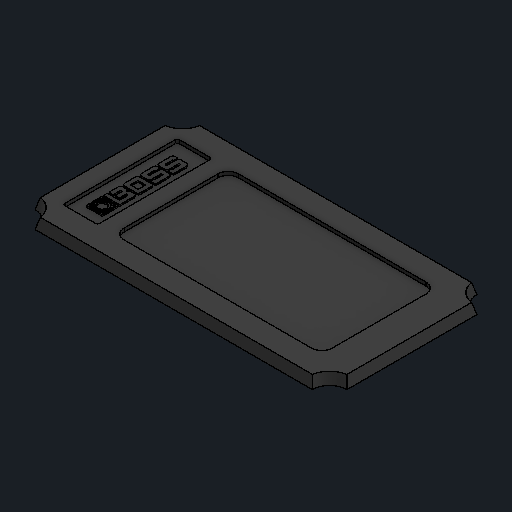
# Autodesk Inventor part: Bottom
Saved by Autodesk Inventor 2026.2 (Build 302298000, 298)
## iProperties
Created: 2015-05-06
Part Number: Bottom
Material: Rubber
Document SubType Name: Modeling
Designer: Philip
Density: 0.93 g/cm^3
Appearance: Rubber - Black
Author: Philip
Autodesk Inventor part; units mm, degrees
(part 1 of 2)
ref_plane "YZ Plane" through (0, 0, 0) normal (1, 0, 0) x (0, 1, 0)
ref_plane "XZ Plane" through (0, 0, 0) normal (0, 1, 0) x (-1, 0, 0)
ref_plane "XY Plane" through (0, 0, 0) normal (0, 0, 1) x (1, 0, 0)
sketch "Sketch1" plane through (0, 0, 0) normal (0, 1, 0) x (-1, 0, 0)
  line L0 (-50.8, 30.1625) -> (50.8, 30.1625)
  line L1 (57.15, 23.8125) -> (57.15, -23.8125)
  line L2 (50.8, -30.1625) -> (-50.8, -30.1625)
  line L3 (-57.15, -23.8125) -> (-57.15, 23.8125)
  arc A0 (57.15, -23.8125) -> (50.8, -30.1625) centre (57.15, -30.1625) ccw
  arc A1 (50.8, 30.1625) -> (57.15, 23.8125) centre (57.15, 30.1625) ccw
  arc A2 (-57.15, 23.8125) -> (-50.8, 30.1625) centre (-57.15, 30.1625) ccw
  arc A3 (-50.8, -30.1625) -> (-57.15, -23.8125) centre (-57.15, -30.1625) ccw
  point P0 (0, 0)
  dimension "d2" = 30.1625
  dimension "d3" = 57.15
  dimension "d4" = 12.7
  dimension "d5" = 12.7
  dimension "d6" = 12.7
  dimension "d7" = 12.7
  dimension "d8" = 60.325
  dimension "d9" = 114.3
  constraints: 8 end point, 8 point on circle, 8 point on line, 4 centre point, 2 parallel, 1 horizontal, 1 perpendicular
  measures "d2" distance from line of L2 point (0, 0)
  measures "d3" distance from line of L3 point (0, 0)
  measures "d4" diameter of A1
  measures "d5" diameter of A0
  measures "d6" diameter of A3
  measures "d7" diameter of A2
  measures "d8" distance between parallel lines of L0 L2
  measures "d9" distance between parallel lines of L3 L1
extrude "Extrusion1" add sketch "Sketch1" along normal blind 3.81 draft -15
sketch "Sketch2" plane through (0, 3.81, 0) normal (0, 1, 0) x (1, 0, 0)
  line L0 (41.275, -20.955) -> (-27.305, -20.955)
  line L1 (-31.115, -17.145) -> (-31.115, 17.145)
  line L2 (-27.305, 20.955) -> (41.275, 20.955)
  line L3 (45.085, 17.145) -> (45.085, -17.145)
  line L4 (57.15, -23.8125) -> (57.15, 23.8125) projected
  arc A0 (-31.115, -17.145) -> (-27.305, -20.955) centre (-27.305, -17.145) ccw
  arc A1 (-27.305, 20.955) -> (-31.115, 17.145) centre (-27.305, 17.145) ccw
  arc A2 (45.085, 17.145) -> (41.275, 20.955) centre (41.275, 17.145) ccw
  arc A3 (41.275, -20.955) -> (45.085, -17.145) centre (41.275, -17.145) ccw
  point P0 (0, 0)
  dimension "d12" = 41.91
  dimension "d13" = 76.2
  dimension "d14" = 12.065
  dimension "d15" = 20.955
  dimension "d16" = 3.81
  constraints: 8 end point, 8 point on circle, 8 tangent, 4 centre point, 3 equal radius, 2 parallel, 1 horizontal, 1 perpendicular
  measures "d12" distance between parallel lines of L0 L2
  measures "d13" distance between parallel lines of L3 L1
  measures "d14" distance between parallel lines of L4 L3
  measures "d15" distance from line of L2 point (0, 0)
  measures "d16" radius of A0
extrude "Extrusion2" cut sketch "Sketch2" against normal blind 1.27
sketch "Sketch3" plane through (0, 3.81, 0) normal (0, 1, 0) x (1, 0, 0)
  line L0 (-37.084, -20.955) -> (-49.784, -20.955)
  line L1 (-49.784, -20.955) -> (-49.784, 20.955)
  line L2 (-49.784, 20.955) -> (-37.084, 20.955)
  line L3 (-37.084, 20.955) -> (-37.084, -20.955)
  line L4 (-57.15, 23.8125) -> (-57.15, -23.8125) projected
  point P0 (0, 0)
  dimension "d19" = 12.7
  dimension "d20" = 41.91
  dimension "d21" = 20.955
  dimension "d22" = 7.366
  constraints: 8 end point, 2 parallel, 1 horizontal, 1 perpendicular
  measures "d19" distance of L0.start L0.end
  measures "d20" distance of L0.end L1.end
  measures "d21" distance from line of L2 point (0, 0)
  measures "d22" distance between parallel lines of L1 L4
extrude "Extrusion3" cut sketch "Sketch3" against normal blind 1.27
fillet "Fillet1" radius 0.762 4 edges at (-49.784, 3.175, -20.955) (-37.084, 3.175, -20.955) (-49.784, 3.175, 20.955) (-37.084, 3.175, 20.955)
sketch "Sketch4" plane through (0, 2.54, 0) normal (0, 1, 0) x (1, 0, 0)
  spline S0 degree 3 poles (-43.0316, -4.1814) (-43.5525, -3.6848) (-43.6527, -3.6265) (-44.0797, -3.6102) (-44.3848, -3.5985) (-44.6906, -3.5918) (-44.9957, -3.5992) (-45.6406, -3.6147) (-46.0256, -4.0139) (-46.0266, -4.6593) (-46.0282, -5.6176) (-46.0275, -6.5759) (-46.0263, -7.5343) (-46.0262, -7.6258) (-46.0164, -7.7174) (-46.0106, -7.8159) (-45.4978, -7.8159) (-45.0079, -7.8159) (-44.4878, -7.8159) (-44.4878, -7.695) (-44.4878, -7.5924) (-44.4878, -7.4897) (-44.4878, -6.8157) (-44.4745, -6.1413) (-44.4937, -5.4679) (-44.5024, -5.1624) (-44.3483, -5.1292) (-44.1066, -5.1197) (-43.8293, -5.1088) (-43.8019, -5.2605) (-43.8044, -5.4778) (-43.8114, -6.0675) (-43.8068, -6.6573) (-43.8068, -7.247) (-43.8068, -7.4322) (-43.8068, -7.6174) (-43.8068, -7.8036) (-43.2785, -7.8036) (-42.7976, -7.8036) (-42.2829, -7.8036) (-42.2829, -7.6745) (-42.2829, -7.5617) (-42.2829, -7.449) (-42.2829, -6.8066) (-42.274, -6.1641) (-42.2871, -5.5219) (-42.2927, -5.2482) (-42.1967, -5.1507) (-41.9196, -5.1546) (-41.6546, -5.1583) (-41.5384, -5.2321) (-41.5425, -5.5161) (-41.555, -6.3794) (-41.5609, -7.2434) (-41.5398, -8.1064) (-41.532, -8.4253) (-41.6497, -8.4936) (-41.9412, -8.4905) (-43.1731, -8.4775) (-44.4054, -8.485) (-45.6375, -8.485) (-45.76, -8.485) (-45.8825, -8.485) (-46.0162, -8.485) (-46.0162, -8.9723) (-46.0162, -9.4197) (-46.0162, -9.8818) (-44.0372, -9.8818) (-42.0744, -9.8818) (-40.0967, -9.8818) (-40.0917, -9.7942) (-40.084, -9.7227) (-40.084, -9.6513) (-40.0833, -7.9136) (-40.0822, -6.176) (-40.0843, -4.4384) (-40.085, -3.9463) (-40.3224, -3.6749) (-40.8182, -3.6299) (-41.1422, -3.6005) (-41.4707, -3.6245) (-41.796, -3.605) (-42.3094, -3.5743) (-42.7245, -3.7436) (-43.0316, -4.1814) knots 0 0 0 0 1 1 1 2 2 2 3 3 3 4 4 4 5 5 5 6 6 6 7 7 7 8 8 8 9 9 9 10 10 10 11 11 11 12 12 12 13 13 13 14 14 14 15 15 15 16 16 16 17 17 17 18 18 18 19 19 19 20 20 20 21 21 21 22 22 22 23 23 23 24 24 24 25 25 25 26 26 26 27 27 27 28 28 28 28
  line L0 (-43.0316, -4.1814) -> (-43.5525, -3.6848) construction
  line L1 (-43.5525, -3.6848) -> (-43.6527, -3.6265) construction
  line L2 (-43.6527, -3.6265) -> (-44.0797, -3.6102) construction
  line L3 (-44.0797, -3.6102) -> (-44.3848, -3.5985) construction
  line L4 (-44.3848, -3.5985) -> (-44.6906, -3.5918) construction
  line L5 (-44.6906, -3.5918) -> (-44.9957, -3.5992) construction
  line L6 (-44.9957, -3.5992) -> (-45.6406, -3.6147) construction
  line L7 (-45.6406, -3.6147) -> (-46.0256, -4.0139) construction
  line L8 (-46.0256, -4.0139) -> (-46.0266, -4.6593) construction
  line L9 (-46.0266, -4.6593) -> (-46.0282, -5.6176) construction
  line L10 (-46.0282, -5.6176) -> (-46.0275, -6.5759) construction
  line L11 (-46.0275, -6.5759) -> (-46.0263, -7.5343) construction
  line L12 (-46.0263, -7.5343) -> (-46.0262, -7.6258) construction
  line L13 (-46.0262, -7.6258) -> (-46.0164, -7.7174) construction
  line L14 (-46.0164, -7.7174) -> (-46.0106, -7.8159) construction
  line L15 (-46.0106, -7.8159) -> (-45.4978, -7.8159) construction
  line L16 (-45.4978, -7.8159) -> (-45.0079, -7.8159) construction
  line L17 (-45.0079, -7.8159) -> (-44.4878, -7.8159) construction
  line L18 (-44.4878, -7.8159) -> (-44.4878, -7.695) construction
  line L19 (-44.4878, -7.695) -> (-44.4878, -7.5924) construction
  line L20 (-44.4878, -7.5924) -> (-44.4878, -7.4897) construction
  line L21 (-44.4878, -7.4897) -> (-44.4878, -6.8157) construction
  line L22 (-44.4878, -6.8157) -> (-44.4745, -6.1413) construction
  line L23 (-44.4745, -6.1413) -> (-44.4937, -5.4679) construction
  line L24 (-44.4937, -5.4679) -> (-44.5024, -5.1624) construction
  line L25 (-44.5024, -5.1624) -> (-44.3483, -5.1292) construction
  line L26 (-44.3483, -5.1292) -> (-44.1066, -5.1197) construction
  line L27 (-44.1066, -5.1197) -> (-43.8293, -5.1088) construction
  line L28 (-43.8293, -5.1088) -> (-43.8019, -5.2605) construction
  line L29 (-43.8019, -5.2605) -> (-43.8044, -5.4778) construction
  line L30 (-43.8044, -5.4778) -> (-43.8114, -6.0675) construction
  line L31 (-43.8114, -6.0675) -> (-43.8068, -6.6573) construction
  line L32 (-43.8068, -6.6573) -> (-43.8068, -7.247) construction
  line L33 (-43.8068, -7.247) -> (-43.8068, -7.4322) construction
  line L34 (-43.8068, -7.4322) -> (-43.8068, -7.6174) construction
  line L35 (-43.8068, -7.6174) -> (-43.8068, -7.8036) construction
  line L36 (-43.8068, -7.8036) -> (-43.2785, -7.8036) construction
  line L37 (-43.2785, -7.8036) -> (-42.7976, -7.8036) construction
  line L38 (-42.7976, -7.8036) -> (-42.2829, -7.8036) construction
  line L39 (-42.2829, -7.8036) -> (-42.2829, -7.6745) construction
  line L40 (-42.2829, -7.6745) -> (-42.2829, -7.5617) construction
  line L41 (-42.2829, -7.5617) -> (-42.2829, -7.449) construction
  line L42 (-42.2829, -7.449) -> (-42.2829, -6.8066) construction
  line L43 (-42.2829, -6.8066) -> (-42.274, -6.1641) construction
  line L44 (-42.274, -6.1641) -> (-42.2871, -5.5219) construction
  line L45 (-42.2871, -5.5219) -> (-42.2927, -5.2482) construction
  line L46 (-42.2927, -5.2482) -> (-42.1967, -5.1507) construction
  line L47 (-42.1967, -5.1507) -> (-41.9196, -5.1546) construction
  line L48 (-41.9196, -5.1546) -> (-41.6546, -5.1583) construction
  line L49 (-41.6546, -5.1583) -> (-41.5384, -5.2321) construction
  line L50 (-41.5384, -5.2321) -> (-41.5425, -5.5161) construction
  line L51 (-41.5425, -5.5161) -> (-41.555, -6.3794) construction
  line L52 (-41.555, -6.3794) -> (-41.5609, -7.2434) construction
  line L53 (-41.5609, -7.2434) -> (-41.5398, -8.1064) construction
  line L54 (-41.5398, -8.1064) -> (-41.532, -8.4253) construction
  line L55 (-41.532, -8.4253) -> (-41.6497, -8.4936) construction
  line L56 (-41.6497, -8.4936) -> (-41.9412, -8.4905) construction
  line L57 (-41.9412, -8.4905) -> (-43.1731, -8.4775) construction
  line L58 (-43.1731, -8.4775) -> (-44.4054, -8.485) construction
  line L59 (-44.4054, -8.485) -> (-45.6375, -8.485) construction
  line L60 (-45.6375, -8.485) -> (-45.76, -8.485) construction
  line L61 (-45.76, -8.485) -> (-45.8825, -8.485) construction
  line L62 (-45.8825, -8.485) -> (-46.0162, -8.485) construction
  line L63 (-46.0162, -8.485) -> (-46.0162, -8.9723) construction
  line L64 (-46.0162, -8.9723) -> (-46.0162, -9.4197) construction
  line L65 (-46.0162, -9.4197) -> (-46.0162, -9.8818) construction
  line L66 (-46.0162, -9.8818) -> (-44.0372, -9.8818) construction
  line L67 (-44.0372, -9.8818) -> (-42.0744, -9.8818) construction
  line L68 (-42.0744, -9.8818) -> (-40.0967, -9.8818) construction
  line L69 (-40.0967, -9.8818) -> (-40.0917, -9.7942) construction
  line L70 (-40.0917, -9.7942) -> (-40.084, -9.7227) construction
  line L71 (-40.084, -9.7227) -> (-40.084, -9.6513) construction
  line L72 (-40.084, -9.6513) -> (-40.0833, -7.9136) construction
  line L73 (-40.0833, -7.9136) -> (-40.0822, -6.176) construction
  line L74 (-40.0822, -6.176) -> (-40.0843, -4.4384) construction
  line L75 (-40.0843, -4.4384) -> (-40.085, -3.9463) construction
  line L76 (-40.085, -3.9463) -> (-40.3224, -3.6749) construction
  line L77 (-40.3224, -3.6749) -> (-40.8182, -3.6299) construction
  line L78 (-40.8182, -3.6299) -> (-41.1422, -3.6005) construction
  line L79 (-41.1422, -3.6005) -> (-41.4707, -3.6245) construction
  line L80 (-41.4707, -3.6245) -> (-41.796, -3.605) construction
  line L81 (-41.796, -3.605) -> (-42.3094, -3.5743) construction
  line L82 (-42.3094, -3.5743) -> (-42.7245, -3.7436) construction
  line L83 (-42.7245, -3.7436) -> (-43.0316, -4.1814) construction
  spline S1 degree 3 poles (-41.9941, 11.0766) (-41.9941, 10.8187) (-41.9941, 10.5987) (-41.9941, 10.3787) (-41.9941, 10.1518) (-41.9941, 9.925) (-41.9941, 9.6815) (-41.6533, 9.6815) (-41.3595, 9.6806) (-41.0658, 9.6817) (-40.358, 9.6843) (-40.0852, 9.9506) (-40.0841, 10.6497) (-40.0819, 11.9656) (-40.0821, 13.2814) (-40.084, 14.5973) (-40.0849, 15.2273) (-40.4452, 15.5915) (-41.0823, 15.5992) (-41.6612, 15.6063) (-42.2402, 15.6014) (-42.8192, 15.6009) (-43.5958, 15.6003) (-43.9177, 15.2847) (-43.9194, 14.5159) (-43.9216, 13.5159) (-43.9232, 12.5158) (-43.9177, 11.5158) (-43.9164, 11.2866) (-43.9415, 11.142) (-44.2378, 11.1432) (-44.5385, 11.1444) (-44.5824, 11.2777) (-44.5783, 11.5302) (-44.5668, 12.2458) (-44.5744, 12.9617) (-44.5742, 13.6776) (-44.5742, 13.8772) (-44.6059, 14.0899) (-44.324, 14.1464) (-44.2864, 14.1539) (-44.2408, 14.242) (-44.24, 14.2934) (-44.2332, 14.712) (-44.2362, 15.1308) (-44.2362, 15.5802) (-44.5687, 15.5802) (-44.872, 15.5857) (-45.1751, 15.5791) (-45.7941, 15.5656) (-46.0271, 15.3344) (-46.0299, 14.7056) (-46.036, 13.3266) (-46.0363, 11.9476) (-46.03, 10.5686) (-46.0272, 9.9562) (-45.7484, 9.682) (-45.1408, 9.6764) (-44.5092, 9.6705) (-43.8776, 9.6742) (-43.246, 9.6749) (-42.5345, 9.6757) (-42.2996, 9.9071) (-42.2982, 10.6156) (-42.2961, 11.6578) (-42.2923, 12.7) (-42.3015, 13.742) (-42.3037, 13.9919) (-42.2666, 14.1221) (-41.9632, 14.1258) (-41.6382, 14.1298) (-41.6399, 13.9603) (-41.6416, 13.7311) (-41.6471, 12.9838) (-41.6478, 12.2363) (-41.6413, 11.489) (-41.6391, 11.2445) (-41.6482, 11.0291) (-41.9941, 11.0766) knots 0 0 0 0 1 1 1 2 2 2 3 3 3 4 4 4 5 5 5 6 6 6 7 7 7 8 8 8 9 9 9 10 10 10 11 11 11 12 12 12 13 13 13 14 14 14 15 15 15 16 16 16 17 17 17 18 18 18 19 19 19 20 20 20 21 21 21 22 22 22 23 23 23 24 24 24 25 25 25 26 26 26 26
  line L84 (-41.9941, 11.0766) -> (-41.9941, 10.8187) construction
  line L85 (-41.9941, 10.8187) -> (-41.9941, 10.5987) construction
  line L86 (-41.9941, 10.5987) -> (-41.9941, 10.3787) construction
  line L87 (-41.9941, 10.3787) -> (-41.9941, 10.1518) construction
  line L88 (-41.9941, 10.1518) -> (-41.9941, 9.925) construction
  line L89 (-41.9941, 9.925) -> (-41.9941, 9.6815) construction
  line L90 (-41.9941, 9.6815) -> (-41.6533, 9.6815) construction
  line L91 (-41.6533, 9.6815) -> (-41.3595, 9.6806) construction
  line L92 (-41.3595, 9.6806) -> (-41.0658, 9.6817) construction
  line L93 (-41.0658, 9.6817) -> (-40.358, 9.6843) construction
  line L94 (-40.358, 9.6843) -> (-40.0852, 9.9506) construction
  line L95 (-40.0852, 9.9506) -> (-40.0841, 10.6497) construction
  line L96 (-40.0841, 10.6497) -> (-40.0819, 11.9656) construction
  line L97 (-40.0819, 11.9656) -> (-40.0821, 13.2814) construction
  line L98 (-40.0821, 13.2814) -> (-40.084, 14.5973) construction
  line L99 (-40.084, 14.5973) -> (-40.0849, 15.2273) construction
  line L100 (-40.0849, 15.2273) -> (-40.4452, 15.5915) construction
  line L101 (-40.4452, 15.5915) -> (-41.0823, 15.5992) construction
  line L102 (-41.0823, 15.5992) -> (-41.6612, 15.6063) construction
  line L103 (-41.6612, 15.6063) -> (-42.2402, 15.6014) construction
  line L104 (-42.2402, 15.6014) -> (-42.8192, 15.6009) construction
  line L105 (-42.8192, 15.6009) -> (-43.5958, 15.6003) construction
  line L106 (-43.5958, 15.6003) -> (-43.9177, 15.2847) construction
  line L107 (-43.9177, 15.2847) -> (-43.9194, 14.5159) construction
  line L108 (-43.9194, 14.5159) -> (-43.9216, 13.5159) construction
  line L109 (-43.9216, 13.5159) -> (-43.9232, 12.5158) construction
  line L110 (-43.9232, 12.5158) -> (-43.9177, 11.5158) construction
  line L111 (-43.9177, 11.5158) -> (-43.9164, 11.2866) construction
  line L112 (-43.9164, 11.2866) -> (-43.9415, 11.142) construction
  line L113 (-43.9415, 11.142) -> (-44.2378, 11.1432) construction
  line L114 (-44.2378, 11.1432) -> (-44.5385, 11.1444) construction
  line L115 (-44.5385, 11.1444) -> (-44.5824, 11.2777) construction
  line L116 (-44.5824, 11.2777) -> (-44.5783, 11.5302) construction
  line L117 (-44.5783, 11.5302) -> (-44.5668, 12.2458) construction
  line L118 (-44.5668, 12.2458) -> (-44.5744, 12.9617) construction
  line L119 (-44.5744, 12.9617) -> (-44.5742, 13.6776) construction
  line L120 (-44.5742, 13.6776) -> (-44.5742, 13.8772) construction
  line L121 (-44.5742, 13.8772) -> (-44.6059, 14.0899) construction
  line L122 (-44.6059, 14.0899) -> (-44.324, 14.1464) construction
  line L123 (-44.324, 14.1464) -> (-44.2864, 14.1539) construction
  line L124 (-44.2864, 14.1539) -> (-44.2408, 14.242) construction
  line L125 (-44.2408, 14.242) -> (-44.24, 14.2934) construction
  line L126 (-44.24, 14.2934) -> (-44.2332, 14.712) construction
  line L127 (-44.2332, 14.712) -> (-44.2362, 15.1308) construction
  line L128 (-44.2362, 15.1308) -> (-44.2362, 15.5802) construction
  line L129 (-44.2362, 15.5802) -> (-44.5687, 15.5802) construction
  line L130 (-44.5687, 15.5802) -> (-44.872, 15.5857) construction
  line L131 (-44.872, 15.5857) -> (-45.1751, 15.5791) construction
  line L132 (-45.1751, 15.5791) -> (-45.7941, 15.5656) construction
  line L133 (-45.7941, 15.5656) -> (-46.0271, 15.3344) construction
  line L134 (-46.0271, 15.3344) -> (-46.0299, 14.7056) construction
  line L135 (-46.0299, 14.7056) -> (-46.036, 13.3266) construction
  line L136 (-46.036, 13.3266) -> (-46.0363, 11.9476) construction
  line L137 (-46.0363, 11.9476) -> (-46.03, 10.5686) construction
  line L138 (-46.03, 10.5686) -> (-46.0272, 9.9562) construction
  line L139 (-46.0272, 9.9562) -> (-45.7484, 9.682) construction
  line L140 (-45.7484, 9.682) -> (-45.1408, 9.6764) construction
  line L141 (-45.1408, 9.6764) -> (-44.5092, 9.6705) construction
  line L142 (-44.5092, 9.6705) -> (-43.8776, 9.6742) construction
  line L143 (-43.8776, 9.6742) -> (-43.246, 9.6749) construction
  line L144 (-43.246, 9.6749) -> (-42.5345, 9.6757) construction
  line L145 (-42.5345, 9.6757) -> (-42.2996, 9.9071) construction
  line L146 (-42.2996, 9.9071) -> (-42.2982, 10.6156) construction
  line L147 (-42.2982, 10.6156) -> (-42.2961, 11.6578) construction
  line L148 (-42.2961, 11.6578) -> (-42.2923, 12.7) construction
  line L149 (-42.2923, 12.7) -> (-42.3015, 13.742) construction
  line L150 (-42.3015, 13.742) -> (-42.3037, 13.9919) construction
  line L151 (-42.3037, 13.9919) -> (-42.2666, 14.1221) construction
  line L152 (-42.2666, 14.1221) -> (-41.9632, 14.1258) construction
  line L153 (-41.9632, 14.1258) -> (-41.6382, 14.1298) construction
  line L154 (-41.6382, 14.1298) -> (-41.6399, 13.9603) construction
  line L155 (-41.6399, 13.9603) -> (-41.6416, 13.7311) construction
  line L156 (-41.6416, 13.7311) -> (-41.6471, 12.9838) construction
  line L157 (-41.6471, 12.9838) -> (-41.6478, 12.2363) construction
  line L158 (-41.6478, 12.2363) -> (-41.6413, 11.489) construction
  line L159 (-41.6413, 11.489) -> (-41.6391, 11.2445) construction
  line L160 (-41.6391, 11.2445) -> (-41.6482, 11.0291) construction
  line L161 (-41.6482, 11.0291) -> (-41.9941, 11.0766) construction
  spline S2 degree 3 poles (-44.2474, 9.1251) (-44.547, 9.1251) (-44.8291, 9.1265) (-45.1112, 9.1248) (-45.7896, 9.1207) (-46.0284, 8.8905) (-46.0307, 8.2153) (-46.0352, 6.8567) (-46.0356, 5.498) (-46.0307, 4.1394) (-46.0284, 3.4861) (-45.7637, 3.2212) (-45.1064, 3.2123) (-44.4746, 3.2036) (-43.8425, 3.2081) (-43.2106, 3.2105) (-42.5495, 3.2131) (-42.3, 3.4632) (-42.2984, 4.1292) (-42.2958, 5.193) (-42.2917, 6.2568) (-42.3018, 7.3204) (-42.3043, 7.5774) (-42.2269, 7.6704) (-41.9588, 7.6723) (-41.6931, 7.6742) (-41.6386, 7.5646) (-41.6409, 7.3338) (-41.6487, 6.565) (-41.6531, 5.7959) (-41.6385, 5.0274) (-41.6335, 4.7662) (-41.6973, 4.6013) (-41.9779, 4.5999) (-41.9779, 4.1358) (-41.9779, 3.6971) (-41.9779, 3.2234) (-41.6393, 3.2234) (-41.3159, 3.2184) (-40.9928, 3.2245) (-40.3657, 3.2364) (-40.0868, 3.5132) (-40.0849, 4.1372) (-40.0807, 5.4853) (-40.0812, 6.8335) (-40.0845, 8.1816) (-40.0859, 8.7551) (-40.457, 9.1274) (-41.0323, 9.1333) (-41.6325, 9.1395) (-42.2347, 9.106) (-42.8328, 9.1423) (-43.5554, 9.186) (-43.9453, 8.7218) (-43.9268, 8.0419) (-43.8999, 7.0526) (-43.9247, 6.062) (-43.9167, 5.0721) (-43.9148, 4.8256) (-43.9485, 4.6864) (-44.2553, 4.6898) (-44.5478, 4.6931) (-44.5801, 4.8245) (-44.5774, 5.059) (-44.5689, 5.7857) (-44.5689, 6.5125) (-44.5772, 7.2392) (-44.5801, 7.4848) (-44.5559, 7.6884) (-44.2474, 7.6919) (-44.2474, 8.1746) (-44.2474, 8.6351) (-44.2474, 9.1251) knots 0 0 0 0 1 1 1 2 2 2 3 3 3 4 4 4 5 5 5 6 6 6 7 7 7 8 8 8 9 9 9 10 10 10 11 11 11 12 12 12 13 13 13 14 14 14 15 15 15 16 16 16 17 17 17 18 18 18 19 19 19 20 20 20 21 21 21 22 22 22 23 23 23 24 24 24 24
  line L162 (-44.2474, 9.1251) -> (-44.547, 9.1251) construction
  line L163 (-44.547, 9.1251) -> (-44.8291, 9.1265) construction
  line L164 (-44.8291, 9.1265) -> (-45.1112, 9.1248) construction
  line L165 (-45.1112, 9.1248) -> (-45.7896, 9.1207) construction
  line L166 (-45.7896, 9.1207) -> (-46.0284, 8.8905) construction
  line L167 (-46.0284, 8.8905) -> (-46.0307, 8.2153) construction
  line L168 (-46.0307, 8.2153) -> (-46.0352, 6.8567) construction
  line L169 (-46.0352, 6.8567) -> (-46.0356, 5.498) construction
  line L170 (-46.0356, 5.498) -> (-46.0307, 4.1394) construction
  line L171 (-46.0307, 4.1394) -> (-46.0284, 3.4861) construction
  line L172 (-46.0284, 3.4861) -> (-45.7637, 3.2212) construction
  line L173 (-45.7637, 3.2212) -> (-45.1064, 3.2123) construction
  line L174 (-45.1064, 3.2123) -> (-44.4746, 3.2036) construction
  line L175 (-44.4746, 3.2036) -> (-43.8425, 3.2081) construction
  line L176 (-43.8425, 3.2081) -> (-43.2106, 3.2105) construction
  line L177 (-43.2106, 3.2105) -> (-42.5495, 3.2131) construction
  line L178 (-42.5495, 3.2131) -> (-42.3, 3.4632) construction
  line L179 (-42.3, 3.4632) -> (-42.2984, 4.1292) construction
  line L180 (-42.2984, 4.1292) -> (-42.2958, 5.193) construction
  line L181 (-42.2958, 5.193) -> (-42.2917, 6.2568) construction
  line L182 (-42.2917, 6.2568) -> (-42.3018, 7.3204) construction
  line L183 (-42.3018, 7.3204) -> (-42.3043, 7.5774) construction
  line L184 (-42.3043, 7.5774) -> (-42.2269, 7.6704) construction
  line L185 (-42.2269, 7.6704) -> (-41.9588, 7.6723) construction
  line L186 (-41.9588, 7.6723) -> (-41.6931, 7.6742) construction
  line L187 (-41.6931, 7.6742) -> (-41.6386, 7.5646) construction
  line L188 (-41.6386, 7.5646) -> (-41.6409, 7.3338) construction
  line L189 (-41.6409, 7.3338) -> (-41.6487, 6.565) construction
  line L190 (-41.6487, 6.565) -> (-41.6531, 5.7959) construction
  line L191 (-41.6531, 5.7959) -> (-41.6385, 5.0274) construction
  line L192 (-41.6385, 5.0274) -> (-41.6335, 4.7662) construction
  line L193 (-41.6335, 4.7662) -> (-41.6973, 4.6013) construction
  line L194 (-41.6973, 4.6013) -> (-41.9779, 4.5999) construction
  line L195 (-41.9779, 4.5999) -> (-41.9779, 4.1358) construction
  line L196 (-41.9779, 4.1358) -> (-41.9779, 3.6971) construction
  line L197 (-41.9779, 3.6971) -> (-41.9779, 3.2234) construction
  line L198 (-41.9779, 3.2234) -> (-41.6393, 3.2234) construction
  line L199 (-41.6393, 3.2234) -> (-41.3159, 3.2184) construction
  line L200 (-41.3159, 3.2184) -> (-40.9928, 3.2245) construction
  line L201 (-40.9928, 3.2245) -> (-40.3657, 3.2364) construction
  line L202 (-40.3657, 3.2364) -> (-40.0868, 3.5132) construction
  line L203 (-40.0868, 3.5132) -> (-40.0849, 4.1372) construction
  line L204 (-40.0849, 4.1372) -> (-40.0807, 5.4853) construction
  line L205 (-40.0807, 5.4853) -> (-40.0812, 6.8335) construction
  line L206 (-40.0812, 6.8335) -> (-40.0845, 8.1816) construction
  line L207 (-40.0845, 8.1816) -> (-40.0859, 8.7551) construction
  line L208 (-40.0859, 8.7551) -> (-40.457, 9.1274) construction
  line L209 (-40.457, 9.1274) -> (-41.0323, 9.1333) construction
  line L210 (-41.0323, 9.1333) -> (-41.6325, 9.1395) construction
  line L211 (-41.6325, 9.1395) -> (-42.2347, 9.106) construction
  line L212 (-42.2347, 9.106) -> (-42.8328, 9.1423) construction
  line L213 (-42.8328, 9.1423) -> (-43.5554, 9.186) construction
  line L214 (-43.5554, 9.186) -> (-43.9453, 8.7218) construction
  line L215 (-43.9453, 8.7218) -> (-43.9268, 8.0419) construction
  line L216 (-43.9268, 8.0419) -> (-43.8999, 7.0526) construction
  line L217 (-43.8999, 7.0526) -> (-43.9247, 6.062) construction
  line L218 (-43.9247, 6.062) -> (-43.9167, 5.0721) construction
  line L219 (-43.9167, 5.0721) -> (-43.9148, 4.8256) construction
  line L220 (-43.9148, 4.8256) -> (-43.9485, 4.6864) construction
  line L221 (-43.9485, 4.6864) -> (-44.2553, 4.6898) construction
  line L222 (-44.2553, 4.6898) -> (-44.5478, 4.6931) construction
  line L223 (-44.5478, 4.6931) -> (-44.5801, 4.8245) construction
  line L224 (-44.5801, 4.8245) -> (-44.5774, 5.059) construction
  line L225 (-44.5774, 5.059) -> (-44.5689, 5.7857) construction
  line L226 (-44.5689, 5.7857) -> (-44.5689, 6.5125) construction
  line L227 (-44.5689, 6.5125) -> (-44.5772, 7.2392) construction
  line L228 (-44.5772, 7.2392) -> (-44.5801, 7.4848) construction
  line L229 (-44.5801, 7.4848) -> (-44.5559, 7.6884) construction
  line L230 (-44.5559, 7.6884) -> (-44.2474, 7.6919) construction
  line L231 (-44.2474, 7.6919) -> (-44.2474, 8.1746) construction
  line L232 (-44.2474, 8.1746) -> (-44.2474, 8.6351) construction
  line L233 (-44.2474, 8.6351) -> (-44.2474, 9.1251) construction
  spline S3 degree 3 poles (-43.0206, -3.0328) (-42.3474, -3.0328) (-41.6742, -3.0392) (-41.0012, -3.031) (-40.3593, -3.0232) (-40.0862, -2.7432) (-40.0845, -2.0983) (-40.0811, -0.8257) (-40.0811, 0.447) (-40.0845, 1.7196) (-40.0861, 2.3514) (-40.3992, 2.6624) (-41.0405, 2.6645) (-42.3657, 2.6688) (-43.6909, 2.6685) (-45.0162, 2.6647) (-45.631, 2.6629) (-46.031, 2.2514) (-46.0319, 1.6283) (-46.0336, 0.4082) (-46.0341, -0.8118) (-46.0317, -2.0319) (-46.0304, -2.6732) (-45.6795, -3.0278) (-45.04, -3.0321) (-44.3669, -3.0367) (-43.6937, -3.0331) (-43.0206, -3.0328) knots 0 0 0 0 1 1 1 2 2 2 3 3 3 4 4 4 5 5 5 6 6 6 7 7 7 8 8 8 9 9 9 9
  line L234 (-43.0206, -3.0328) -> (-42.3474, -3.0328) construction
  line L235 (-42.3474, -3.0328) -> (-41.6742, -3.0392) construction
  line L236 (-41.6742, -3.0392) -> (-41.0012, -3.031) construction
  line L237 (-41.0012, -3.031) -> (-40.3593, -3.0232) construction
  line L238 (-40.3593, -3.0232) -> (-40.0862, -2.7432) construction
  line L239 (-40.0862, -2.7432) -> (-40.0845, -2.0983) construction
  line L240 (-40.0845, -2.0983) -> (-40.0811, -0.8257) construction
  line L241 (-40.0811, -0.8257) -> (-40.0811, 0.447) construction
  line L242 (-40.0811, 0.447) -> (-40.0845, 1.7196) construction
  line L243 (-40.0845, 1.7196) -> (-40.0861, 2.3514) construction
  line L244 (-40.0861, 2.3514) -> (-40.3992, 2.6624) construction
  line L245 (-40.3992, 2.6624) -> (-41.0405, 2.6645) construction
  line L246 (-41.0405, 2.6645) -> (-42.3657, 2.6688) construction
  line L247 (-42.3657, 2.6688) -> (-43.6909, 2.6685) construction
  line L248 (-43.6909, 2.6685) -> (-45.0162, 2.6647) construction
  line L249 (-45.0162, 2.6647) -> (-45.631, 2.6629) construction
  line L250 (-45.631, 2.6629) -> (-46.031, 2.2514) construction
  line L251 (-46.031, 2.2514) -> (-46.0319, 1.6283) construction
  line L252 (-46.0319, 1.6283) -> (-46.0336, 0.4082) construction
  line L253 (-46.0336, 0.4082) -> (-46.0341, -0.8118) construction
  line L254 (-46.0341, -0.8118) -> (-46.0317, -2.0319) construction
  line L255 (-46.0317, -2.0319) -> (-46.0304, -2.6732) construction
  line L256 (-46.0304, -2.6732) -> (-45.6795, -3.0278) construction
  line L257 (-45.6795, -3.0278) -> (-45.04, -3.0321) construction
  line L258 (-45.04, -3.0321) -> (-44.3669, -3.0367) construction
  line L259 (-44.3669, -3.0367) -> (-43.6937, -3.0331) construction
  line L260 (-43.6937, -3.0331) -> (-43.0206, -3.0328) construction
  spline S4 degree 3 poles (-46.0019, -16.1978) (-44.0121, -16.1978) (-42.0581, -16.1978) (-40.0922, -16.1978) (-40.0922, -14.2497) (-40.0922, -12.3189) (-40.0922, -10.378) (-42.0717, -10.378) (-44.032, -10.378) (-45.9953, -10.378) (-45.9953, -11.7534) (-45.9953, -13.1051) (-45.9953, -14.4608) (-45.5366, -14.4608) (-45.1001, -14.4608) (-44.6407, -14.4608) (-44.6407, -14.0643) (-44.6169, -13.6853) (-44.6453, -13.3103) (-44.7205, -12.3188) (-43.9795, -11.8681) (-43.3179, -11.7553) (-42.3658, -11.593) (-41.4438, -12.2885) (-41.3775, -13.241) (-41.3239, -14.0121) (-41.8875, -14.9147) (-43.006, -14.882) (-43.8893, -14.8563) (-44.7741, -14.8763) (-45.6582, -14.8776) (-45.7697, -14.8778) (-45.8811, -14.8876) (-46.0019, -14.8935) (-46.0019, -15.3412) (-46.0019, -15.7578) (-46.0019, -16.1978) knots 0 0 0 0 1 1 1 2 2 2 3 3 3 4 4 4 5 5 5 6 6 6 7 7 7 8 8 8 9 9 9 10 10 10 11 11 11 12 12 12 12
  line L261 (-46.0019, -16.1978) -> (-44.0121, -16.1978) construction
  line L262 (-44.0121, -16.1978) -> (-42.0581, -16.1978) construction
  line L263 (-42.0581, -16.1978) -> (-40.0922, -16.1978) construction
  line L264 (-40.0922, -16.1978) -> (-40.0922, -14.2497) construction
  line L265 (-40.0922, -14.2497) -> (-40.0922, -12.3189) construction
  line L266 (-40.0922, -12.3189) -> (-40.0922, -10.378) construction
  line L267 (-40.0922, -10.378) -> (-42.0717, -10.378) construction
  line L268 (-42.0717, -10.378) -> (-44.032, -10.378) construction
  line L269 (-44.032, -10.378) -> (-45.9953, -10.378) construction
  line L270 (-45.9953, -10.378) -> (-45.9953, -11.7534) construction
  line L271 (-45.9953, -11.7534) -> (-45.9953, -13.1051) construction
  line L272 (-45.9953, -13.1051) -> (-45.9953, -14.4608) construction
  line L273 (-45.9953, -14.4608) -> (-45.5366, -14.4608) construction
  line L274 (-45.5366, -14.4608) -> (-45.1001, -14.4608) construction
  line L275 (-45.1001, -14.4608) -> (-44.6407, -14.4608) construction
  line L276 (-44.6407, -14.4608) -> (-44.6407, -14.0643) construction
  line L277 (-44.6407, -14.0643) -> (-44.6169, -13.6853) construction
  line L278 (-44.6169, -13.6853) -> (-44.6453, -13.3103) construction
  line L279 (-44.6453, -13.3103) -> (-44.7205, -12.3188) construction
  line L280 (-44.7205, -12.3188) -> (-43.9795, -11.8681) construction
  line L281 (-43.9795, -11.8681) -> (-43.3179, -11.7553) construction
  line L282 (-43.3179, -11.7553) -> (-42.3658, -11.593) construction
  line L283 (-42.3658, -11.593) -> (-41.4438, -12.2885) construction
  line L284 (-41.4438, -12.2885) -> (-41.3775, -13.241) construction
  line L285 (-41.3775, -13.241) -> (-41.3239, -14.0121) construction
  line L286 (-41.3239, -14.0121) -> (-41.8875, -14.9147) construction
  line L287 (-41.8875, -14.9147) -> (-43.006, -14.882) construction
  line L288 (-43.006, -14.882) -> (-43.8893, -14.8563) construction
  line L289 (-43.8893, -14.8563) -> (-44.7741, -14.8763) construction
  line L290 (-44.7741, -14.8763) -> (-45.6582, -14.8776) construction
  line L291 (-45.6582, -14.8776) -> (-45.7697, -14.8778) construction
  line L292 (-45.7697, -14.8778) -> (-45.8811, -14.8876) construction
  line L293 (-45.8811, -14.8876) -> (-46.0019, -14.8935) construction
  line L294 (-46.0019, -14.8935) -> (-46.0019, -15.3412) construction
  line L295 (-46.0019, -15.3412) -> (-46.0019, -15.7578) construction
  line L296 (-46.0019, -15.7578) -> (-46.0019, -16.1978) construction
  spline S5 degree 3 poles (-43.0316, -4.1814) (-42.7245, -3.7436) (-42.3094, -3.5743) (-41.796, -3.605) (-41.4707, -3.6245) (-41.1422, -3.6005) (-40.8182, -3.6299) (-40.3224, -3.6749) (-40.085, -3.9463) (-40.0843, -4.4384) (-40.0822, -6.176) (-40.0833, -7.9136) (-40.084, -9.6513) (-40.084, -9.7227) (-40.0917, -9.7942) (-40.0967, -9.8818) (-42.0744, -9.8818) (-44.0372, -9.8818) (-46.0162, -9.8818) (-46.0162, -9.4197) (-46.0162, -8.9723) (-46.0162, -8.485) (-45.8825, -8.485) (-45.76, -8.485) (-45.6375, -8.485) (-44.4054, -8.485) (-43.1731, -8.4775) (-41.9412, -8.4905) (-41.6497, -8.4936) (-41.532, -8.4253) (-41.5398, -8.1064) (-41.5609, -7.2434) (-41.555, -6.3794) (-41.5425, -5.5161) (-41.5384, -5.2321) (-41.6546, -5.1583) (-41.9196, -5.1546) (-42.1967, -5.1507) (-42.2927, -5.2482) (-42.2871, -5.5219) (-42.274, -6.1641) (-42.2829, -6.8066) (-42.2829, -7.449) (-42.2829, -7.5617) (-42.2829, -7.6745) (-42.2829, -7.8036) (-42.7976, -7.8036) (-43.2785, -7.8036) (-43.8068, -7.8036) (-43.8068, -7.6174) (-43.8068, -7.4322) (-43.8068, -7.247) (-43.8068, -6.6573) (-43.8114, -6.0675) (-43.8044, -5.4778) (-43.8019, -5.2605) (-43.8293, -5.1088) (-44.1066, -5.1197) (-44.3483, -5.1292) (-44.5024, -5.1624) (-44.4937, -5.4679) (-44.4745, -6.1413) (-44.4878, -6.8157) (-44.4878, -7.4897) (-44.4878, -7.5924) (-44.4878, -7.695) (-44.4878, -7.8159) (-45.0079, -7.8159) (-45.4978, -7.8159) (-46.0106, -7.8159) (-46.0164, -7.7174) (-46.0262, -7.6258) (-46.0263, -7.5343) (-46.0275, -6.5759) (-46.0282, -5.6176) (-46.0266, -4.6593) (-46.0256, -4.0139) (-45.6406, -3.6147) (-44.9957, -3.5992) (-44.6906, -3.5918) (-44.3848, -3.5985) (-44.0797, -3.6102) (-43.6527, -3.6265) (-43.5525, -3.6848) (-43.0316, -4.1814) knots 0 0 0 0 1 1 1 2 2 2 3 3 3 4 4 4 5 5 5 6 6 6 7 7 7 8 8 8 9 9 9 10 10 10 11 11 11 12 12 12 13 13 13 14 14 14 15 15 15 16 16 16 17 17 17 18 18 18 19 19 19 20 20 20 21 21 21 22 22 22 23 23 23 24 24 24 25 25 25 26 26 26 27 27 27 28 28 28 28
  line L297 (-43.0316, -4.1814) -> (-42.7245, -3.7436) construction
  line L298 (-42.7245, -3.7436) -> (-42.3094, -3.5743) construction
  line L299 (-42.3094, -3.5743) -> (-41.796, -3.605) construction
  line L300 (-41.796, -3.605) -> (-41.4707, -3.6245) construction
  line L301 (-41.4707, -3.6245) -> (-41.1422, -3.6005) construction
  line L302 (-41.1422, -3.6005) -> (-40.8182, -3.6299) construction
  line L303 (-40.8182, -3.6299) -> (-40.3224, -3.6749) construction
  line L304 (-40.3224, -3.6749) -> (-40.085, -3.9463) construction
  line L305 (-40.085, -3.9463) -> (-40.0843, -4.4384) construction
  line L306 (-40.0843, -4.4384) -> (-40.0822, -6.176) construction
  line L307 (-40.0822, -6.176) -> (-40.0833, -7.9136) construction
  line L308 (-40.0833, -7.9136) -> (-40.084, -9.6513) construction
  line L309 (-40.084, -9.6513) -> (-40.084, -9.7227) construction
  line L310 (-40.084, -9.7227) -> (-40.0917, -9.7942) construction
  line L311 (-40.0917, -9.7942) -> (-40.0967, -9.8818) construction
  line L312 (-40.0967, -9.8818) -> (-42.0744, -9.8818) construction
  line L313 (-42.0744, -9.8818) -> (-44.0372, -9.8818) construction
  line L314 (-44.0372, -9.8818) -> (-46.0162, -9.8818) construction
  line L315 (-46.0162, -9.8818) -> (-46.0162, -9.4197) construction
  line L316 (-46.0162, -9.4197) -> (-46.0162, -8.9723) construction
  line L317 (-46.0162, -8.9723) -> (-46.0162, -8.485) construction
  line L318 (-46.0162, -8.485) -> (-45.8825, -8.485) construction
  line L319 (-45.8825, -8.485) -> (-45.76, -8.485) construction
  line L320 (-45.76, -8.485) -> (-45.6375, -8.485) construction
  line L321 (-45.6375, -8.485) -> (-44.4054, -8.485) construction
  line L322 (-44.4054, -8.485) -> (-43.1731, -8.4775) construction
  line L323 (-43.1731, -8.4775) -> (-41.9412, -8.4905) construction
  line L324 (-41.9412, -8.4905) -> (-41.6497, -8.4936) construction
  line L325 (-41.6497, -8.4936) -> (-41.532, -8.4253) construction
  line L326 (-41.532, -8.4253) -> (-41.5398, -8.1064) construction
  line L327 (-41.5398, -8.1064) -> (-41.5609, -7.2434) construction
  line L328 (-41.5609, -7.2434) -> (-41.555, -6.3794) construction
  line L329 (-41.555, -6.3794) -> (-41.5425, -5.5161) construction
  line L330 (-41.5425, -5.5161) -> (-41.5384, -5.2321) construction
  line L331 (-41.5384, -5.2321) -> (-41.6546, -5.1583) construction
  line L332 (-41.6546, -5.1583) -> (-41.9196, -5.1546) construction
  line L333 (-41.9196, -5.1546) -> (-42.1967, -5.1507) construction
  line L334 (-42.1967, -5.1507) -> (-42.2927, -5.2482) construction
  line L335 (-42.2927, -5.2482) -> (-42.2871, -5.5219) construction
  line L336 (-42.2871, -5.5219) -> (-42.274, -6.1641) construction
  line L337 (-42.274, -6.1641) -> (-42.2829, -6.8066) construction
  line L338 (-42.2829, -6.8066) -> (-42.2829, -7.449) construction
  line L339 (-42.2829, -7.449) -> (-42.2829, -7.5617) construction
  line L340 (-42.2829, -7.5617) -> (-42.2829, -7.6745) construction
  line L341 (-42.2829, -7.6745) -> (-42.2829, -7.8036) construction
  line L342 (-42.2829, -7.8036) -> (-42.7976, -7.8036) construction
  line L343 (-42.7976, -7.8036) -> (-43.2785, -7.8036) construction
  line L344 (-43.2785, -7.8036) -> (-43.8068, -7.8036) construction
  line L345 (-43.8068, -7.8036) -> (-43.8068, -7.6174) construction
  line L346 (-43.8068, -7.6174) -> (-43.8068, -7.4322) construction
  line L347 (-43.8068, -7.4322) -> (-43.8068, -7.247) construction
  line L348 (-43.8068, -7.247) -> (-43.8068, -6.6573) construction
  line L349 (-43.8068, -6.6573) -> (-43.8114, -6.0675) construction
  line L350 (-43.8114, -6.0675) -> (-43.8044, -5.4778) construction
  line L351 (-43.8044, -5.4778) -> (-43.8019, -5.2605) construction
  line L352 (-43.8019, -5.2605) -> (-43.8293, -5.1088) construction
  line L353 (-43.8293, -5.1088) -> (-44.1066, -5.1197) construction
  line L354 (-44.1066, -5.1197) -> (-44.3483, -5.1292) construction
  line L355 (-44.3483, -5.1292) -> (-44.5024, -5.1624) construction
  line L356 (-44.5024, -5.1624) -> (-44.4937, -5.4679) construction
  line L357 (-44.4937, -5.4679) -> (-44.4745, -6.1413) construction
  line L358 (-44.4745, -6.1413) -> (-44.4878, -6.8157) construction
  line L359 (-44.4878, -6.8157) -> (-44.4878, -7.4897) construction
  line L360 (-44.4878, -7.4897) -> (-44.4878, -7.5924) construction
  line L361 (-44.4878, -7.5924) -> (-44.4878, -7.695) construction
  line L362 (-44.4878, -7.695) -> (-44.4878, -7.8159) construction
  line L363 (-44.4878, -7.8159) -> (-45.0079, -7.8159) construction
  line L364 (-45.0079, -7.8159) -> (-45.4978, -7.8159) construction
  line L365 (-45.4978, -7.8159) -> (-46.0106, -7.8159) construction
  line L366 (-46.0106, -7.8159) -> (-46.0164, -7.7174) construction
  line L367 (-46.0164, -7.7174) -> (-46.0262, -7.6258) construction
  line L368 (-46.0262, -7.6258) -> (-46.0263, -7.5343) construction
  line L369 (-46.0263, -7.5343) -> (-46.0275, -6.5759) construction
  line L370 (-46.0275, -6.5759) -> (-46.0282, -5.6176) construction
  line L371 (-46.0282, -5.6176) -> (-46.0266, -4.6593) construction
  line L372 (-46.0266, -4.6593) -> (-46.0256, -4.0139) construction
  line L373 (-46.0256, -4.0139) -> (-45.6406, -3.6147) construction
  line L374 (-45.6406, -3.6147) -> (-44.9957, -3.5992) construction
  line L375 (-44.9957, -3.5992) -> (-44.6906, -3.5918) construction
  line L376 (-44.6906, -3.5918) -> (-44.3848, -3.5985) construction
  line L377 (-44.3848, -3.5985) -> (-44.0797, -3.6102) construction
  line L378 (-44.0797, -3.6102) -> (-43.6527, -3.6265) construction
  line L379 (-43.6527, -3.6265) -> (-43.5525, -3.6848) construction
  line L380 (-43.5525, -3.6848) -> (-43.0316, -4.1814) construction
  spline S6 degree 3 poles (-41.9941, 11.0766) (-41.6482, 11.0291) (-41.6391, 11.2445) (-41.6413, 11.489) (-41.6478, 12.2363) (-41.6471, 12.9838) (-41.6416, 13.7311) (-41.6399, 13.9603) (-41.6382, 14.1298) (-41.9632, 14.1258) (-42.2666, 14.1221) (-42.3037, 13.9919) (-42.3015, 13.742) (-42.2923, 12.7) (-42.2961, 11.6578) (-42.2982, 10.6156) (-42.2996, 9.9071) (-42.5345, 9.6757) (-43.246, 9.6749) (-43.8776, 9.6742) (-44.5092, 9.6705) (-45.1408, 9.6764) (-45.7484, 9.682) (-46.0272, 9.9562) (-46.03, 10.5686) (-46.0363, 11.9476) (-46.036, 13.3266) (-46.0299, 14.7056) (-46.0271, 15.3344) (-45.7941, 15.5656) (-45.1751, 15.5791) (-44.872, 15.5857) (-44.5687, 15.5802) (-44.2362, 15.5802) (-44.2362, 15.1308) (-44.2332, 14.712) (-44.24, 14.2934) (-44.2408, 14.242) (-44.2864, 14.1539) (-44.324, 14.1464) (-44.6059, 14.0899) (-44.5742, 13.8772) (-44.5742, 13.6776) (-44.5744, 12.9617) (-44.5668, 12.2458) (-44.5783, 11.5302) (-44.5824, 11.2777) (-44.5385, 11.1444) (-44.2378, 11.1432) (-43.9415, 11.142) (-43.9164, 11.2866) (-43.9177, 11.5158) (-43.9232, 12.5158) (-43.9216, 13.5159) (-43.9194, 14.5159) (-43.9177, 15.2847) (-43.5958, 15.6003) (-42.8192, 15.6009) (-42.2402, 15.6014) (-41.6612, 15.6063) (-41.0823, 15.5992) (-40.4452, 15.5915) (-40.0849, 15.2273) (-40.084, 14.5973) (-40.0821, 13.2814) (-40.0819, 11.9656) (-40.0841, 10.6497) (-40.0852, 9.9506) (-40.358, 9.6843) (-41.0658, 9.6817) (-41.3595, 9.6806) (-41.6533, 9.6815) (-41.9941, 9.6815) (-41.9941, 9.925) (-41.9941, 10.1518) (-41.9941, 10.3787) (-41.9941, 10.5987) (-41.9941, 10.8187) (-41.9941, 11.0766) knots 0 0 0 0 1 1 1 2 2 2 3 3 3 4 4 4 5 5 5 6 6 6 7 7 7 8 8 8 9 9 9 10 10 10 11 11 11 12 12 12 13 13 13 14 14 14 15 15 15 16 16 16 17 17 17 18 18 18 19 19 19 20 20 20 21 21 21 22 22 22 23 23 23 24 24 24 25 25 25 26 26 26 26
  line L381 (-41.9941, 11.0766) -> (-41.6482, 11.0291) construction
  line L382 (-41.6482, 11.0291) -> (-41.6391, 11.2445) construction
  line L383 (-41.6391, 11.2445) -> (-41.6413, 11.489) construction
  line L384 (-41.6413, 11.489) -> (-41.6478, 12.2363) construction
  line L385 (-41.6478, 12.2363) -> (-41.6471, 12.9838) construction
  line L386 (-41.6471, 12.9838) -> (-41.6416, 13.7311) construction
  line L387 (-41.6416, 13.7311) -> (-41.6399, 13.9603) construction
  line L388 (-41.6399, 13.9603) -> (-41.6382, 14.1298) construction
  line L389 (-41.6382, 14.1298) -> (-41.9632, 14.1258) construction
  line L390 (-41.9632, 14.1258) -> (-42.2666, 14.1221) construction
  line L391 (-42.2666, 14.1221) -> (-42.3037, 13.9919) construction
  line L392 (-42.3037, 13.9919) -> (-42.3015, 13.742) construction
  line L393 (-42.3015, 13.742) -> (-42.2923, 12.7) construction
  line L394 (-42.2923, 12.7) -> (-42.2961, 11.6578) construction
  line L395 (-42.2961, 11.6578) -> (-42.2982, 10.6156) construction
  line L396 (-42.2982, 10.6156) -> (-42.2996, 9.9071) construction
  line L397 (-42.2996, 9.9071) -> (-42.5345, 9.6757) construction
  line L398 (-42.5345, 9.6757) -> (-43.246, 9.6749) construction
  line L399 (-43.246, 9.6749) -> (-43.8776, 9.6742) construction
  line L400 (-43.8776, 9.6742) -> (-44.5092, 9.6705) construction
  line L401 (-44.5092, 9.6705) -> (-45.1408, 9.6764) construction
  line L402 (-45.1408, 9.6764) -> (-45.7484, 9.682) construction
  line L403 (-45.7484, 9.682) -> (-46.0272, 9.9562) construction
  line L404 (-46.0272, 9.9562) -> (-46.03, 10.5686) construction
  line L405 (-46.03, 10.5686) -> (-46.0363, 11.9476) construction
  line L406 (-46.0363, 11.9476) -> (-46.036, 13.3266) construction
  line L407 (-46.036, 13.3266) -> (-46.0299, 14.7056) construction
  line L408 (-46.0299, 14.7056) -> (-46.0271, 15.3344) construction
  line L409 (-46.0271, 15.3344) -> (-45.7941, 15.5656) construction
  line L410 (-45.7941, 15.5656) -> (-45.1751, 15.5791) construction
  line L411 (-45.1751, 15.5791) -> (-44.872, 15.5857) construction
  line L412 (-44.872, 15.5857) -> (-44.5687, 15.5802) construction
  line L413 (-44.5687, 15.5802) -> (-44.2362, 15.5802) construction
  line L414 (-44.2362, 15.5802) -> (-44.2362, 15.1308) construction
  line L415 (-44.2362, 15.1308) -> (-44.2332, 14.712) construction
  line L416 (-44.2332, 14.712) -> (-44.24, 14.2934) construction
  line L417 (-44.24, 14.2934) -> (-44.2408, 14.242) construction
  line L418 (-44.2408, 14.242) -> (-44.2864, 14.1539) construction
  line L419 (-44.2864, 14.1539) -> (-44.324, 14.1464) construction
  line L420 (-44.324, 14.1464) -> (-44.6059, 14.0899) construction
  line L421 (-44.6059, 14.0899) -> (-44.5742, 13.8772) construction
  line L422 (-44.5742, 13.8772) -> (-44.5742, 13.6776) construction
  line L423 (-44.5742, 13.6776) -> (-44.5744, 12.9617) construction
  line L424 (-44.5744, 12.9617) -> (-44.5668, 12.2458) construction
  line L425 (-44.5668, 12.2458) -> (-44.5783, 11.5302) construction
  line L426 (-44.5783, 11.5302) -> (-44.5824, 11.2777) construction
  line L427 (-44.5824, 11.2777) -> (-44.5385, 11.1444) construction
  line L428 (-44.5385, 11.1444) -> (-44.2378, 11.1432) construction
  line L429 (-44.2378, 11.1432) -> (-43.9415, 11.142) construction
  line L430 (-43.9415, 11.142) -> (-43.9164, 11.2866) construction
  line L431 (-43.9164, 11.2866) -> (-43.9177, 11.5158) construction
  line L432 (-43.9177, 11.5158) -> (-43.9232, 12.5158) construction
  line L433 (-43.9232, 12.5158) -> (-43.9216, 13.5159) construction
  line L434 (-43.9216, 13.5159) -> (-43.9194, 14.5159) construction
  line L435 (-43.9194, 14.5159) -> (-43.9177, 15.2847) construction
  line L436 (-43.9177, 15.2847) -> (-43.5958, 15.6003) construction
  line L437 (-43.5958, 15.6003) -> (-42.8192, 15.6009) construction
  line L438 (-42.8192, 15.6009) -> (-42.2402, 15.6014) construction
  line L439 (-42.2402, 15.6014) -> (-41.6612, 15.6063) construction
  line L440 (-41.6612, 15.6063) -> (-41.0823, 15.5992) construction
  line L441 (-41.0823, 15.5992) -> (-40.4452, 15.5915) construction
  line L442 (-40.4452, 15.5915) -> (-40.0849, 15.2273) construction
  line L443 (-40.0849, 15.2273) -> (-40.084, 14.5973) construction
  line L444 (-40.084, 14.5973) -> (-40.0821, 13.2814) construction
  line L445 (-40.0821, 13.2814) -> (-40.0819, 11.9656) construction
  line L446 (-40.0819, 11.9656) -> (-40.0841, 10.6497) construction
  line L447 (-40.0841, 10.6497) -> (-40.0852, 9.9506) construction
  line L448 (-40.0852, 9.9506) -> (-40.358, 9.6843) construction
  line L449 (-40.358, 9.6843) -> (-41.0658, 9.6817) construction
  line L450 (-41.0658, 9.6817) -> (-41.3595, 9.6806) construction
  line L451 (-41.3595, 9.6806) -> (-41.6533, 9.6815) construction
  line L452 (-41.6533, 9.6815) -> (-41.9941, 9.6815) construction
  line L453 (-41.9941, 9.6815) -> (-41.9941, 9.925) construction
  line L454 (-41.9941, 9.925) -> (-41.9941, 10.1518) construction
  line L455 (-41.9941, 10.1518) -> (-41.9941, 10.3787) construction
  line L456 (-41.9941, 10.3787) -> (-41.9941, 10.5987) construction
  line L457 (-41.9941, 10.5987) -> (-41.9941, 10.8187) construction
  line L458 (-41.9941, 10.8187) -> (-41.9941, 11.0766) construction
  spline S7 degree 3 poles (-44.2474, 9.1251) (-44.2474, 8.6351) (-44.2474, 8.1746) (-44.2474, 7.6919) (-44.5559, 7.6884) (-44.5801, 7.4848) (-44.5772, 7.2392) (-44.5689, 6.5125) (-44.5689, 5.7857) (-44.5774, 5.059) (-44.5801, 4.8245) (-44.5478, 4.6931) (-44.2553, 4.6898) (-43.9485, 4.6864) (-43.9148, 4.8256) (-43.9167, 5.0721) (-43.9247, 6.062) (-43.8999, 7.0526) (-43.9268, 8.0419) (-43.9453, 8.7218) (-43.5554, 9.186) (-42.8328, 9.1423) (-42.2347, 9.106) (-41.6325, 9.1395) (-41.0323, 9.1333) (-40.457, 9.1274) (-40.0859, 8.7551) (-40.0845, 8.1816) (-40.0812, 6.8335) (-40.0807, 5.4853) (-40.0849, 4.1372) (-40.0868, 3.5132) (-40.3657, 3.2364) (-40.9928, 3.2245) (-41.3159, 3.2184) (-41.6393, 3.2234) (-41.9779, 3.2234) (-41.9779, 3.6971) (-41.9779, 4.1358) (-41.9779, 4.5999) (-41.6973, 4.6013) (-41.6335, 4.7662) (-41.6385, 5.0274) (-41.6531, 5.7959) (-41.6487, 6.565) (-41.6409, 7.3338) (-41.6386, 7.5646) (-41.6931, 7.6742) (-41.9588, 7.6723) (-42.2269, 7.6704) (-42.3043, 7.5774) (-42.3018, 7.3204) (-42.2917, 6.2568) (-42.2958, 5.193) (-42.2984, 4.1292) (-42.3, 3.4632) (-42.5495, 3.2131) (-43.2106, 3.2105) (-43.8425, 3.2081) (-44.4746, 3.2036) (-45.1064, 3.2123) (-45.7637, 3.2212) (-46.0284, 3.4861) (-46.0307, 4.1394) (-46.0356, 5.498) (-46.0352, 6.8567) (-46.0307, 8.2153) (-46.0284, 8.8905) (-45.7896, 9.1207) (-45.1112, 9.1248) (-44.8291, 9.1265) (-44.547, 9.1251) (-44.2474, 9.1251) knots 0 0 0 0 1 1 1 2 2 2 3 3 3 4 4 4 5 5 5 6 6 6 7 7 7 8 8 8 9 9 9 10 10 10 11 11 11 12 12 12 13 13 13 14 14 14 15 15 15 16 16 16 17 17 17 18 18 18 19 19 19 20 20 20 21 21 21 22 22 22 23 23 23 24 24 24 24
  line L459 (-44.2474, 9.1251) -> (-44.2474, 8.6351) construction
  line L460 (-44.2474, 8.6351) -> (-44.2474, 8.1746) construction
  line L461 (-44.2474, 8.1746) -> (-44.2474, 7.6919) construction
  line L462 (-44.2474, 7.6919) -> (-44.5559, 7.6884) construction
  line L463 (-44.5559, 7.6884) -> (-44.5801, 7.4848) construction
  line L464 (-44.5801, 7.4848) -> (-44.5772, 7.2392) construction
  line L465 (-44.5772, 7.2392) -> (-44.5689, 6.5125) construction
  line L466 (-44.5689, 6.5125) -> (-44.5689, 5.7857) construction
  line L467 (-44.5689, 5.7857) -> (-44.5774, 5.059) construction
  line L468 (-44.5774, 5.059) -> (-44.5801, 4.8245) construction
  line L469 (-44.5801, 4.8245) -> (-44.5478, 4.6931) construction
  line L470 (-44.5478, 4.6931) -> (-44.2553, 4.6898) construction
  line L471 (-44.2553, 4.6898) -> (-43.9485, 4.6864) construction
  line L472 (-43.9485, 4.6864) -> (-43.9148, 4.8256) construction
  line L473 (-43.9148, 4.8256) -> (-43.9167, 5.0721) construction
  line L474 (-43.9167, 5.0721) -> (-43.9247, 6.062) construction
  line L475 (-43.9247, 6.062) -> (-43.8999, 7.0526) construction
  line L476 (-43.8999, 7.0526) -> (-43.9268, 8.0419) construction
  line L477 (-43.9268, 8.0419) -> (-43.9453, 8.7218) construction
  line L478 (-43.9453, 8.7218) -> (-43.5554, 9.186) construction
  line L479 (-43.5554, 9.186) -> (-42.8328, 9.1423) construction
  line L480 (-42.8328, 9.1423) -> (-42.2347, 9.106) construction
  line L481 (-42.2347, 9.106) -> (-41.6325, 9.1395) construction
  line L482 (-41.6325, 9.1395) -> (-41.0323, 9.1333) construction
  line L483 (-41.0323, 9.1333) -> (-40.457, 9.1274) construction
  line L484 (-40.457, 9.1274) -> (-40.0859, 8.7551) construction
  line L485 (-40.0859, 8.7551) -> (-40.0845, 8.1816) construction
  line L486 (-40.0845, 8.1816) -> (-40.0812, 6.8335) construction
  line L487 (-40.0812, 6.8335) -> (-40.0807, 5.4853) construction
  line L488 (-40.0807, 5.4853) -> (-40.0849, 4.1372) construction
  line L489 (-40.0849, 4.1372) -> (-40.0868, 3.5132) construction
  line L490 (-40.0868, 3.5132) -> (-40.3657, 3.2364) construction
  line L491 (-40.3657, 3.2364) -> (-40.9928, 3.2245) construction
  line L492 (-40.9928, 3.2245) -> (-41.3159, 3.2184) construction
  line L493 (-41.3159, 3.2184) -> (-41.6393, 3.2234) construction
  line L494 (-41.6393, 3.2234) -> (-41.9779, 3.2234) construction
  line L495 (-41.9779, 3.2234) -> (-41.9779, 3.6971) construction
  line L496 (-41.9779, 3.6971) -> (-41.9779, 4.1358) construction
  line L497 (-41.9779, 4.1358) -> (-41.9779, 4.5999) construction
  line L498 (-41.9779, 4.5999) -> (-41.6973, 4.6013) construction
  line L499 (-41.6973, 4.6013) -> (-41.6335, 4.7662) construction
  line L500 (-41.6335, 4.7662) -> (-41.6385, 5.0274) construction
  line L501 (-41.6385, 5.0274) -> (-41.6531, 5.7959) construction
  line L502 (-41.6531, 5.7959) -> (-41.6487, 6.565) construction